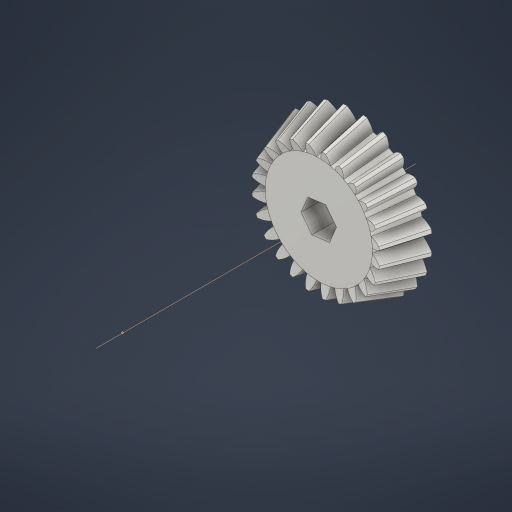
# Autodesk Inventor part: Bevel Gear2
Saved by Autodesk Inventor 2023 (Build 270158000, 158)
## iProperties
CustomPartVersion: 1
Created: 2023-08-11
Part Number: Bevel Gear2
Material: Steel, Mild
Document SubType Name: Modeling
Designer: Izack Waczko
Categories: <?xml version="1.0" encoding="UTF-16"?> <MemberInstance><Categories><FamilyTemplate><FamilyTemplateParameter ValueType="xs:double" Id="1" ObjectReferenceKey="da_z" ObjectType="kUserParameterObject"/><FamilyTemplateParameter ValueType="xs:double" Id="2" ObjectReferenceKey="da_b" ObjectType="kUserParameterObject"/><FamilyTemplateParameter ValueType="xs:double" Id="3" ObjectReferenceKey="da_beta" ObjectType="kUserParameterObject"/><FamilyTemplateParameter ValueType="xs:double" Id="4" ObjectReferenceKey="da_dae" ObjectType="kUserParameterObject"/><FamilyTemplateParameter ValueType="xs:double" Id="5" ObjectReferenceKey="da_ve" ObjectType="kUserParameterObject"/><FamilyTemplateParameter ValueType="xs:double" Id="6" ObjectReferenceKey="da_omega" ObjectType="kUserParameterObject"/><FamilyTemplateParameter ValueType="xs:string" Id="7" ObjectReferenceKey="EAIAABAAAAAAHwAAAAAAAIAAAAAAAAAA" ObjectType="83914240" SubObjectId="SurfaceGeometry"/></FamilyTemplate><ParamToTemplateMap><ParamToTemplate CategoryParameter="//CategoryParameter[@InternalName='046C89C9-8512-4d59-83FE-43B91F4F132A']" TemplateParameter="1"/><ParamToTemplate CategoryParameter="//CategoryParameter[@InternalName='2552DF32-E462-4b46-AEBF-C6C7768E72AC']" TemplateParameter="2"/><ParamToTemplate CategoryParameter="//CategoryParameter[@InternalName='C9EE641D-15FC-4fae-A226-E94C4372FDD7']" TemplateParameter="3"/><ParamToTemplate><ParamToTemplate CategoryParameter="//CategoryParameter[@InternalName='00B6519A-459B-49c7-AD84-2E56D39A5744']" ConstantValue="-0.000000"/></ParamToTemplate><ParamToTemplate><ParamToTemplate CategoryParameter="//CategoryParameter[@InternalName='04B31F0E-C7A6-4894-AA32-9629BEFACF47']" ConstantValue="1.000000"/></ParamToTemplate><ParamToTemplate><ParamToTemplate CategoryParameter="//CategoryParameter[@InternalName='43CBEC2E-7847-49e7-A936-2F7889FCB2D9']" ConstantValue="0.200000"/></ParamToTemplate><ParamToTemplate><ParamToTemplate CategoryParameter="//CategoryParameter[@InternalName='B1EFC894-105D-4ebd-86BF-FA20ED196853']" ConstantValue="0.300000"/></ParamToTemplate><ParamToTemplate><ParamToTemplate CategoryParameter="//CategoryParameter[@InternalName='51175063-3D10-4879-93E8-6246FE8B403D']" ConstantValue="2060000000.000000"/></ParamToTemplate><ParamToTemplate><ParamToTemplate CategoryParameter="//CategoryParameter[@InternalName='A3A52E27-4454-46a9-B0BD-C932399B70AF']" ConstantValue="0.300000"/></ParamToTemplate><ParamToTemplate CategoryParameter="//CategoryParameter[@InternalName='2A200944-5A8C-41ca-B96E-8520D2E510F1']" TemplateParameter="4"/><ParamToTemplate><ParamToTemplate CategoryParameter="//CategoryParameter[@InternalName='1A637F62-92C8-44bc-B81F-10802510B579']" ConstantValue="2.151438"/></ParamToTemplate><ParamToTemplate CategoryParameter="//CategoryParameter[@InternalName='B52DD4BE-6863-48fb-BF58-89EF6F9EC65C']" TemplateParameter="5"/><ParamToTemplate><ParamToTemplate CategoryParameter="//CategoryParameter[@InternalName='3956BFF2-84D2-457d-93C2-9B0613DEBA67']" ConstantValue="3.251142"/></ParamToTemplate><ParamToTemplate CategoryParameter="//CategoryParameter[@InternalName='739CFA02-461B-4bf8-8049-181FCAD8B28F']" TemplateParameter="6"/><ParamToTemplate><ParamToTemplate CategoryParameter="//CategoryParameter[@InternalName='A27E999F-E2CE-4481-8A2A-EBF499C4C3C5']" ConstantValue="-0.000000"/></ParamToTemplate><ParamToTemplate><ParamToTemplate CategoryParameter="//CategoryParameter[@InternalName='9E1B4470-B2D3-4ff1-B813-535BB4CDF51A']" ConstantValue="3520000.000000"/></ParamToTemplate><ParamToTemplate><ParamToTemplate CategoryParameter="//CategoryParameter[@InternalName='F8452263-BFF6-458c-9FB1-07C4B99E95CD']" ConstantValue="11400000.000000"/></ParamToTemplate><ParamToTemplate><ParamToTemplate CategoryParameter="//CategoryParameter[@InternalName='3E3BB259-FD49-497f-8171-6EBC954A3479']" ConstantValue="2.000000"/></ParamToTemplate><ParamToTemplate CategoryParameter="//CategoryParameter[@InternalName='27C3BAF2-7550-4e4b-AE2C-0DB134B7D9B7']" TemplateParameter="7"/></ParamToTemplateMap><Category DisplayName="Gear" InternalName="DC85795E-93AB-48d5-8EEE-5A27447B64BD" Mnemonic="Gear"><CategoryParameter DisplayName="z" InternalName="046C89C9-8512-4d59-83FE-43B91F4F132A" Mnemonic="z"/><CategoryParameter DisplayName="b" InternalName="2552DF32-E462-4b46-AEBF-C6C7768E72AC" Mnemonic="b"/><CategoryParameter DisplayName="||b|" InternalName="C9EE641D-15FC-4fae-A226-E94C4372FDD7" Mnemonic="beta"/><CategoryParameter DisplayName="x" InternalName="00B6519A-459B-49c7-AD84-2E56D39A5744" Mnemonic="x"/><CategoryParameter DisplayName="a*" InternalName="04B31F0E-C7A6-4894-AA32-9629BEFACF47" Mnemonic="a"/><CategoryParameter DisplayName="c*" InternalName="43CBEC2E-7847-49e7-A936-2F7889FCB2D9" Mnemonic="c"/><CategoryParameter DisplayName="r|.f|*" InternalName="B1EFC894-105D-4ebd-86BF-FA20ED196853" Mnemonic="rf"/><CategoryParameter DisplayName="E" InternalName="51175063-3D10-4879-93E8-6246FE8B403D" Mnemonic="E"/><CategoryParameter DisplayName="||m|" InternalName="A3A52E27-4454-46a9-B0BD-C932399B70AF" Mnemonic="mi"/><Category DisplayName="BevelGear" InternalName="0C98F69A-0C2B-4791-B2FE-7691BB227E77" Mnemonic="BevelGear"><CategoryParameter DisplayName="d|.ae|" InternalName="2A200944-5A8C-41ca-B96E-8520D2E510F1" Mnemonic="dae"/><CategoryParameter DisplayName="d|.ai|" InternalName="1A637F62-92C8-44bc-B81F-10802510B579" Mnemonic="dai"/><CategoryParameter DisplayName="A|.e|" InternalName="B52DD4BE-6863-48fb-BF58-89EF6F9EC65C" Mnemonic="ve"/><CategoryParameter DisplayName="A|.i|" InternalName="3956BFF2-84D2-457d-93C2-9B0613DEBA67" Mnemonic="vi"/><CategoryParameter DisplayName="||S|" InternalName="739CFA02-461B-4bf8-8049-181FCAD8B28F" Mnemonic="omega"/><CategoryParameter DisplayName="x|.t|" InternalName="A27E999F-E2CE-4481-8A2A-EBF499C4C3C5" Mnemonic="xt"/><CategoryParameter DisplayName="||s||.Flim|" InternalName="9E1B4470-B2D3-4ff1-B813-535BB4CDF51A" Mnemonic="sFlim"/><CategoryParameter DisplayName="||s||.Hlim|" InternalName="F8452263-BFF6-458c-9FB1-07C4B99E95CD" Mnemonic="sHlim"/><CategoryParameter DisplayName="type" InternalName="3E3BB259-FD49-497f-8171-6EBC954A3479" Mnemonic="type"/><CategoryParameter DisplayName="PitchDiameter" InternalName="27C3BAF2-7550-4e4b-AE2C-0DB134B7D9B7" Mnemonic="IDS_PITCHDIAM"/></Category></Category></Categories></MemberInstance>
Mass: 60.9118 g
Surface Area: 34.3074 cm^2
Volume: 7.7496 cm^3
Density: 7.86 g/cm^3
Appearance: Steel
d48: 0.000 mm
d49: 0.000 mm
d50: 75.00 deg
d52: 0.000 mm
d53: 0.000 mm
d54: 0.00 deg
Author: Izack Waczko
Autodesk Inventor part; units mm, degrees
ref_plane "Mesh Plane2" through (0, 0, 0) normal (0.9914449, 0.1305262, 0) x (0, 0, 1)
sketch "Teeth Body Sketch" plane through (0, 0, 0) normal (1, 0, 0) x (0, 1, 0)
  line L0 (0, 0) -> (10.8519, -39.7993) construction
  line L1 (10.8519, -39.7993) -> (12.9567, -39.159)
  line L2 (12.9567, -39.159) -> (0, 0) construction
  line L3 (12, -39.4501) -> (0, 0) construction
  line L4 (9.0097, -33.043) -> (10.7572, -32.5114)
  line L5 (10.8519, -39.7993) -> (9.0097, -33.043)
  line L6 (12.9567, -39.159) -> (10.7572, -32.5114)
  line L7 (0, -47.5836) -> (0, 7.9306) projected
  line L8 (0, -39.4501) -> (12.9567, -39.4501) construction
  dimension "d0" = 24
  dimension "d1" = 21.7039
  dimension "d2" = 25.9134
  dimension "d3" = 7
  dimension "d4" = 39.159
  constraints: 16 end point, 4 point on line, 3 perpendicular, 2 collinear, 1 horizontal alignment, 1 vertical alignment
  measures "d0" diameter of L3.start L7
  measures "d1" diameter of L0.end L7
  measures "d2" diameter of L1.end L7
  measures "d3" distance between parallel lines of L1 L4
  measures "d4" vertical distance of L1.end L0.start
revolve "Teeth Body" add sketch "Teeth Body Sketch" angle 360 about axis through (0, 0, 0) along (0, 0, 1)
ref_plane "Tooth Plane" through (0, 12, -39.4501) normal (0, -0.2910165, 0.956718) x (1, 0, 0)
sketch "Start Sketch" plane through (0, 12, -39.4501) normal (0, -0.2910165, 0.956718) x (1, 0, 0)
  line L0 (0, -14.7123) -> (0, 4.4007) projected
  arc A0 (-0.4129, -1.464) -> (-1.9249, 1.529) centre (-5.0201, -1.9131) ccw
  arc A1 (1.9249, 1.529) -> (0.4129, -1.464) centre (5.0201, -1.9131) ccw
  line L1 (-0.4129, -1.464) -> (0.4129, -1.464)
  arc A2 (1.9249, 1.529) -> (-1.9249, 1.529) centre (0, -12.5429) ccw
  dimension "d7" = 4.6291
  dimension "d8" = 5.0202
  dimension "d9" = 10.6298
  dimension "d57" = 14.2029
  dimension "d58" = 11.0789
  constraints: 6 point on circle, 3 centre point, 3 symmetric about line, 2 end point, 1 coincident, 1 perpendicular, 1 other
  measures "d7" radius of A0
  measures "d8" horizontal distance of point (0, -12.543) A0.centre
  measures "d9" vertical distance of point (0, -12.543) A0.centre
  measures "d57" radius of A2
  measures "d58" distance from line of A2.centre L1
sketch "End Sketch" plane through (0, 9.9309, -32.6478) normal (0, -0.2910165, 0.956718) x (1, 0, 0)
  line L0 (0, -12.1587) -> (0, 3.6368) projected
  arc A0 (-0.3417, -1.2116) -> (-1.593, 1.2653) centre (-4.1545, -1.5832) ccw
  arc A1 (1.593, 1.2653) -> (0.3417, -1.2116) centre (4.1545, -1.5832) ccw
  line L1 (-0.3417, -1.2116) -> (0.3417, -1.2116)
  arc A2 (1.593, 1.2653) -> (-1.593, 1.2653) centre (0, -10.3801) ccw
  dimension "d12" = 3.8309
  dimension "d15" = 4.1545
  dimension "d16" = 8.7969
  dimension "d59" = 11.7539
  dimension "d60" = 9.1686
  constraints: 6 point on circle, 3 centre point, 3 symmetric about line, 2 end point, 1 coincident, 1 other
  measures "d12" radius of A0
  measures "d15" horizontal distance of A0.centre point (0, -10.38)
  measures "d16" vertical distance of A0.centre point (0, -10.38)
  measures "d59" radius of A2
  measures "d60" distance from line of A2.centre L1
loft "Loft" cut profiles "Start Sketch", "End Sketch"
pattern_circular "Circular Pattern" count 24 over 360 about axis through (0, 0, 0) along (0, 0, 1) of "Loft"
ref_plane "End Plane" through (0, 9.9309, -32.6478) normal (0, -0.2910165, 0.956718) x (1, 0, 0)
sketch3d "3D Sketch Right"
ref_plane "End Plane Right" through (-3.7176, 9.2088, -32.6478) normal (0.1089425, -0.2698558, 0.956718) x (0.9272869, 0.3743515, 0)
sketch "End Sketch Right" plane through (-3.7176, 9.2088, -32.6478) normal (0.1089425, -0.2698558, 0.956718) x (0.9272869, 0.3743515, 0)
  arc A0 (-0.3417, -1.2116) -> (-1.593, 1.2653) centre (-4.1545, -1.5832) ccw
  line L0 (0, -16.4495) -> (0, 7.4497) projected
  arc A1 (1.593, 1.2653) -> (0.3417, -1.2116) centre (4.1545, -1.5832) ccw
  line L1 (-0.3417, -1.2116) -> (0.3417, -1.2116)
  arc A2 (1.593, 1.2653) -> (-1.593, 1.2653) centre (0, -10.3801) ccw
  dimension "d70" = 4.1545
  dimension "d71" = 8.7969
  dimension "d72" = 3.8309
  dimension "d73" = 9.1686
  dimension "d74" = 11.7539
  constraints: 6 point on circle, 3 centre point, 3 symmetric about line, 2 end point, 1 coincident, 1 perpendicular, 1 other
  measures "d70" horizontal distance of A2.centre A0.centre
  measures "d71" vertical distance of point (0, -10.38) A0.centre
  measures "d72" radius of A0
  measures "d73" distance from line of point (0, -10.38) L1
  measures "d74" radius of A2
feature "Loft Right" [suppressed]
pattern_circular "Circular Pattern Right" [suppressed]
sketch3d "3D Sketch Left"
ref_plane "End Plane Left" through (3.7107, 9.2088, -32.644) normal (-0.1087525, -0.2698905, 0.9567299) x (0.92753, -0.3737487, 0)
sketch "End Sketch Left" plane through (3.7107, 9.2088, -32.644) normal (-0.1087525, -0.2698905, 0.9567299) x (0.92753, -0.3737487, 0)
  line L0 (0, -32.6699) -> (0, 15.0517) projected
  arc A0 (-0.3417, -1.2102) -> (-1.593, 1.2667) centre (-4.1545, -1.5818) ccw
  arc A1 (1.593, 1.2667) -> (0.3417, -1.2102) centre (4.1545, -1.5818) ccw
  line L1 (-0.3417, -1.2102) -> (0.3417, -1.2102)
  ellipse E0 centre (0, -9.4601) end of major axis (10.7572, -9.4601) minor radius 10.2917 projected
  arc A2 (1.593, 1.2667) -> (-1.593, 1.2667) centre (0, -10.3788) ccw
  dimension "d56" = 10.2917
  dimension "d30" = 3.8309
  dimension "d31" = 4.1545
  dimension "d32" = 8.7969
  dimension "d61" = 11.7539
  dimension "d62" = 9.1686
  constraints: 6 point on circle, 3 centre point, 3 symmetric about line, 2 end point, 1 coincident, 2 other
  measures "d30" radius of A0
  measures "d31" horizontal distance of point (0, -10.379) A0.centre
  measures "d32" vertical distance of A0.centre point (0, -10.379)
  measures "d61" radius of A2
  measures "d62" distance from line of point (0, -10.379) L1
feature "Loft Left" [suppressed]
pattern_circular "Circular Pattern Left" [suppressed]
sketch "Body Sketch" plane through (0, 0, 0) normal (1, 0, 0) x (0, 1, 0)
  line L0 (0, -41.0082) -> (0, -31.5217) projected
  line L1 (10.8519, -39.7993) -> (9.0097, -33.043) projected
  line L2 (9.0097, -33.043) -> (0, -33.043)
  line L3 (10.8519, -39.7993) -> (0, -39.7993)
  constraints: 4 end point, 2 perpendicular, 2 point on line
revolve "Fix Body" add sketch "Body Sketch" angle 360 about axis through (0, 0, 0) along (0, 0, 1)
sketch "Sketch6" plane through (0, 0, 0) normal (1, 0, 0) x (0, 1, 0)
  line L0 (12, -39.4501) -> (0, 0) projected
  line L1 (0, -47.1793) -> (0, 7.8632) projected
surface revolve "Pitch Diameter" sketch "Sketch6" angle 360 about axis through (0, 0, 0) along (0, 0, 1) shown no curves L0
sketch "Sketch8" plane through (0, 0, -39.7993) normal (0, 0, -1) x (-0.3826834, -0.9238795, 0)
  circle A0 centre (0, 0) radius 2.6 construction
  line L0 (1.5011, 2.6) -> (3.0022, 0)
  line L1 (3.0022, 0) -> (1.5011, -2.6)
  line L2 (1.5011, -2.6) -> (-1.5011, -2.6)
  line L3 (-1.5011, -2.6) -> (-3.0022, 0)
  line L4 (-3.0022, 0) -> (-1.5011, 2.6)
  line L5 (-1.5011, 2.6) -> (1.5011, 2.6)
  point P0 (0, 2.6)
  dimension "d94" = 5.2
  constraints: 12 end point, 2 coincident, 1 midpoint, 1 vertical alignment, 15 other
extrude "Extrusion1" cut sketch "Sketch8" against normal blind 10
equation "\"d0\" = da_de"
equation "\"d1\" = da_dfe"
equation "\"d2\" = da_dae"
equation "\"d3\" = da_b"
equation "\"d4\" = da_ve"
equation "\"d7\" = fd_rr"
equation "\"d8\" = fd_x"
equation "\"d9\" = fd_y"
equation "\"d57\" = 0.5 * fd_dva + 0.3 * da_he"
equation "\"d58\" = 0.5 * fd_dva - 1.12 * da_he"
equation "\"da_teethtype\" = 0"
equation "\"da_b\" = 7"
equation "\"da_de\" = 24"
equation "\"da_dae\" = 25.91344"
equation "\"da_dfe\" = 21.70388"
equation "\"da_le\" = 41.23478"
equation "\"da_omega\" = 75deg"
equation "\"da_beta\" = 0"
equation "\"da_delta\" = 16.918821deg"
equation "\"da_alpha\" = 20deg"
equation "\"da_he\" = 2.2"
equation "\"da_ve\" = 39.15904"
equation "\"da_zv\" = 25.085761"
equation "\"fd_loft\" = da_b + 0.05 * da_he"
equation "\"fd_x\" = fd_x1 + fd_x2"
equation "\"fd_y\" = fd_y1 - fd_y2"
equation "\"fd_dd\" = fd_dva - 0.8 * da_he"
equation "\"da_dvw\" = 25.08576"
equation "\"d11\" = fd_loft"
equation "\"da_dm\" = 21.96288"
equation "\"da_x\" = 0"
equation "\"da_m\" = 1"
equation "\"d50\" = da_omega"
equation "\"fd_rr\" = 4.629048"
equation "\"fd_dva\" = 27.085761"
equation "\"fd_x1\" = 0.793594"
equation "\"fd_x2\" = 4.226554"
equation "\"fd_y1\" = 12.51775"
equation "\"fd_y2\" = 1.887941"
body "Solid1"
body "Srf1"
